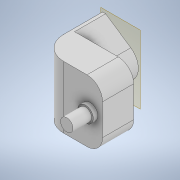
# Autodesk Inventor part: servo_shaft
Saved by Autodesk Inventor 2021 (Build 250183000, 183)
## iProperties
Created: 2021-11-23
Part Number: servo_shaft
Material: Generic
Document SubType Name: Modeling
Designer: techv
Density: 1 g/cm^3
Appearance: Default
Author: techv
Autodesk Inventor part; units mm, degrees
ref_plane "YZ Plane" through (0, 0, 0) normal (1, 0, 0) x (0, 1, 0)
ref_plane "XZ Plane" through (0, 0, 0) normal (0, 1, 0) x (-1, 0, 0)
ref_plane "Work Plane1" through (0, 0, -5) normal (0, 0, 1) x (1, 0, 0)
sketch "Sketch2" plane through (0, 0, -5) normal (0, 0, 1) x (1, 0, 0)
  line L0 (0, 0) -> (16.1462, -10.8737) projected
  line L1 (0, 0) -> (-2, 0) projected
  line L2 (-2, 0) -> (-2, -40) projected
  line L3 (0, -40) -> (-2, -40) projected
  line L4 (16.1462, -29.1263) -> (0, -40) projected
  arc A0 (16.1462, -29.1263) -> (16.1462, -10.8737) centre (10, -20) ccw projected
  circle A1 centre (10, -20) radius 2.5 projected
extrude "Extrusion1" add sketch "Sketch2" along normal blind 20 contours L0 A0 L4 L3 L2 L1 | A1
sketch "Sketch3" plane through (0, 0, 15) normal (0, 0, 1) x (1, 0, 0)
  circle A0 centre (29.9899, -19.3654) radius 4 projected
  line L0 (-2, -40) -> (0, -40) projected
  line L1 (0, -40) -> (16.1462, -29.1263) projected
  arc A1 (16.1462, -29.1263) -> (16.1462, -10.8737) centre (10, -20) ccw projected
  line L2 (16.1462, -10.8737) -> (0, 0) projected
  line L3 (0, 0) -> (-2, 0) projected
  line L4 (-2, 0) -> (-2, -40) projected
  line L5 (0, 0) -> (-2, 0) projected
  line L6 (-2, 0) -> (38, 0)
  line L7 (38, 0) -> (38, -40)
  line L8 (38, -40) -> (-2, -40)
  line L9 (-2, -40) -> (-2, 0)
  point P0 (16.1462, -29.1263)
  point P1 (0, 0)
  point P2 (0, -40)
  dimension "d2" = 40
  dimension "d3" = 40
  constraints: 8 end point, 2 parallel, 1 horizontal, 1 perpendicular
  measures "d2" distance of L7.end L8.end
  measures "d3" distance of L6.end L7.end
ref_plane "Work Plane2" through (-0.7088, -242.7053, 35) normal (0, 0, -1) x (-0.0317282, 0.9994965, 0)
extrude "Extrusion2" add sketch "Sketch3" along normal up to surface (20 mm away) contours A0 | L4 L3 L2 A1 L1 L0 | L1 A1 L2 L6 L7 L8
fillet "Fillet1" radius 15 1 edges at (-2, -20, 35)
fillet "Fillet2" radius 10 2 edges at (38, -40, 25) (38, 0, 25)
sketch "Sketch4" plane through (13, -40, 35) normal (0, 0, 1) x (1, 0, 0)
  circle A0 centre (16.9899, 20.6346) radius 4 projected
  point P0 (-13, 40)
extrude "Extrusion3" add sketch "Sketch4" along normal blind 15
sketch "Sketch5" plane through (13, -40, 35) normal (0, 0, 1) x (1, 0, 0)
  circle A0 centre (16.9899, 20.6346) radius 4 projected
  circle A1 centre (16.9899, 20.6346) radius 5
  point P0 (-13, 40)
  dimension "d10" = 10
  constraints: 1 centre point, 1 coincident
  measures "d10" diameter of A1
extrude "Extrusion4" add sketch "Sketch5" along normal blind 3
body "Solid1"
